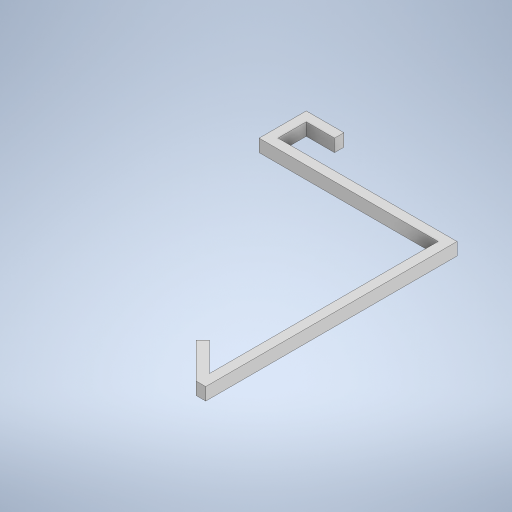
# Autodesk Inventor part: Staffa
Saved by Autodesk Inventor 2024 (Build 280153000, 153)
## iProperties
Created: 2023-12-27
Part Number: Staffa
Material: Generico
Document SubType Name: Sheet Metal
Designer: Leonardo
Density: 1 g/cm^3
Sheet Metal Rule: Default_mm
Appearance: Default
Author: Leonardo
Autodesk Inventor part; units mm, degrees
ref_plane "YZ Plane" through (0, 0, 0) normal (1, 0, 0) x (0, 1, 0)
ref_plane "XZ Plane" through (0, 0, 0) normal (0, 1, 0) x (-1, 0, 0)
ref_plane "XY Plane" through (0, 0, 0) normal (0, 0, 1) x (1, 0, 0)
sketch "Schizzo1" plane through (0, 0, 0) normal (0, 1, 0) x (-1, 0, 0)
  line L0 (300, 0) -> (300, 15)
  line L1 (0, 0) -> (0, 400)
  line L2 (0, 400) -> (15, 400)
  line L3 (15, 400) -> (71.5685, 343.4315)
  line L4 (15, 400) -> (95, 400) construction
  line L5 (71.5685, 343.4315) -> (60.9619, 332.8249)
  line L6 (60.9619, 332.8249) -> (15, 378.7868)
  line L7 (15, 378.7868) -> (15, 15)
  line L8 (300, 15) -> (15, 15)
  line L9 (300, 0) -> (300, -60)
  line L10 (300, -60) -> (240, -60)
  line L11 (240, -60) -> (240, -45)
  line L12 (240, -45) -> (285, -45)
  line L13 (285, -45) -> (285, 0)
  line L14 (285, 0) -> (0, 0)
  dimension "d1" = 15
  dimension "d3" = 400
  dimension "d4" = 15
  dimension "d5" = 80
  dimension "d6" = 45
  dimension "d7" = 15
  dimension "d8" = 60
  dimension "d9" = 60
  dimension "d10" = 15
  dimension "d11" = 45
  constraints: 30 end point, 7 perpendicular, 3 horizontal, 1 equal length, 1 vertical
  measures "d1" distance of L0.end L0.start
  measures "d3" distance of L1.start L1.end
  measures "d4" distance of L1.end L2.end
  measures "d5" distance of L2.end L3.end
  measures "d6" angle of L3 L4
  measures "d7" distance of L3.end L5.end
  measures "d8" distance of L0.start L9.end
  measures "d9" distance of L9.end L10.end
  measures "d10" distance of L10.end L11.end
  measures "d11" distance of L11.end L12.end
extrude "Estrusione1" add sketch "Schizzo1" along normal blind 20
equation "\"RaggioPiega\" = Spessore"
equation "\"LarghezzaScaricoPiega\" = Spessore"
equation "\"ProfonditàScaricoPiega\" = 0.5 * Spessore"
equation "\"DimensioniScaricoAngolo\" = 4 * Spessore"
equation "\"ResiduoMinimo\" = 2 * Spessore"
equation "\"RaggioTransizione\" = RaggioPiega"
equation "\"Dimensione_raggio_Jacobi\" = RaggioPiega"
equation "\"DimensioneGioco\" = Spessore"
equation "\"Spessore\" = 0.5"
